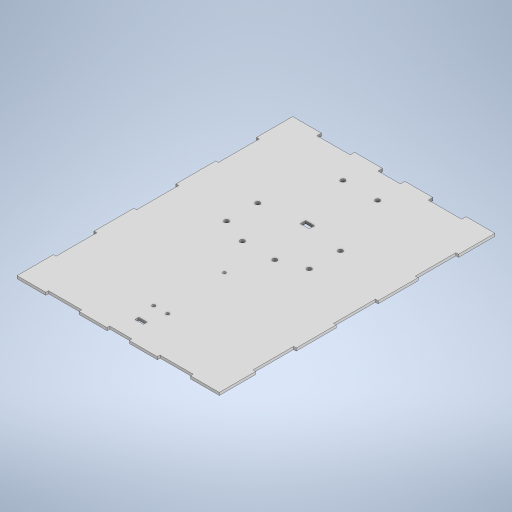
# Autodesk Inventor part: totalPart
Saved by Autodesk Inventor 2023 (Build 270158000, 158)
## iProperties
Created: 2022-11-20
Part Number: totalPart
Material: Generic
Document SubType Name: Modeling
Designer: ADMIN
Density: 1 g/cm^3
Appearance: Default
Author: ADMIN
Autodesk Inventor part; units mm, degrees
ref_plane "YZ Plane" through (0, 0, 0) normal (1, 0, 0) x (0, 1, 0)
ref_plane "XZ Plane" through (0, 0, 0) normal (0, 1, 0) x (-1, 0, 0)
ref_plane "XY Plane" through (0, 0, 0) normal (0, 0, 1) x (1, 0, 0)
sketch "Sketch1" plane through (0, 0, 0) normal (0, 1, 0) x (-1, 0, 0)
  line L0 (128.8824, 62.1664) -> (128.8824, -237.8336)
  line L1 (48.8824, 24.5697) -> (45.8824, 24.5697)
  line L2 (48.8824, -65.4156) -> (45.8824, -65.4156)
  line L3 (48.8824, -20.7764) -> (45.8824, -20.7764)
  line L4 (48.8824, -202.2369) -> (45.8824, -202.2369)
  line L5 (48.8824, -112.2516) -> (45.8824, -112.2516)
  line L6 (48.8824, -156.8908) -> (45.8824, -156.8908)
  line L7 (48.8824, 24.5697) -> (48.8824, 62.1664)
  line L8 (48.8824, 24.5697) -> (48.8824, 65.1664)
  line L9 (48.8824, -65.4156) -> (48.8824, -20.7764)
  line L10 (48.8824, -65.4156) -> (48.8824, -20.7764)
  line L11 (48.8824, -237.8336) -> (48.8824, -202.2369)
  line L12 (48.8824, -156.8908) -> (48.8824, -112.2516)
  line L13 (48.8824, -242.8336) -> (48.8824, -202.2369)
  line L14 (48.8824, -156.8908) -> (48.8824, -112.2516)
  line L15 (45.8824, -20.7764) -> (45.8824, 24.5697)
  line L16 (45.8824, -202.2369) -> (45.8824, -156.8908)
  line L17 (45.8824, -112.2516) -> (45.8824, -65.4156)
  line L18 (-177.1176, 24.5697) -> (-174.1176, 24.5697)
  line L19 (-177.1176, -65.4156) -> (-174.1176, -65.4156)
  line L20 (-177.1176, -20.7764) -> (-174.1176, -20.7764)
  line L21 (-177.1176, -202.2369) -> (-174.1176, -202.2369)
  line L22 (-177.1176, -156.8908) -> (-174.1176, -156.8908)
  line L23 (-177.1176, -112.2516) -> (-174.1176, -112.2516)
  line L24 (-177.1176, 65.1664) -> (-177.1176, 24.5697)
  line L25 (-174.1176, 24.5697) -> (-174.1176, -20.7764)
  line L26 (-177.1176, -20.7764) -> (-177.1176, -65.4156)
  line L27 (-174.1176, -65.4156) -> (-174.1176, -112.2516)
  line L28 (-174.1176, -156.8908) -> (-174.1176, -202.2369)
  line L29 (-177.1176, -112.2516) -> (-177.1176, -156.8908)
  line L30 (-177.1176, -202.2369) -> (-177.1176, -242.8336)
  line L31 (48.8824, -237.8336) -> (48.8824, -242.8336)
  line L32 (128.8824, -242.8336) -> (128.8824, -237.8336)
  line L33 (48.8824, -242.8336) -> (63.8824, -242.8336)
  line L34 (63.8824, -242.8336) -> (63.8824, -237.8336)
  line L35 (63.8824, -237.8336) -> (78.8824, -237.8336)
  line L36 (78.8824, -237.8336) -> (78.8824, -242.8336)
  line L37 (113.8824, -242.8336) -> (113.8824, -237.8336)
  line L38 (98.8824, -237.8336) -> (98.8824, -242.8336)
  line L39 (128.8824, -242.8336) -> (113.8824, -242.8336)
  line L40 (113.8824, -237.8336) -> (98.8824, -237.8336)
  line L41 (78.8824, -237.8336) -> (63.8824, -237.8336)
  line L42 (98.8824, -242.8336) -> (78.8824, -242.8336)
  line L43 (63.8824, -242.8336) -> (48.8824, -242.8336)
  line L44 (63.8824, 65.1664) -> (63.8824, 62.1664)
  line L45 (78.8824, 62.1664) -> (78.8824, 65.1664)
  line L46 (98.8824, 62.1664) -> (98.8824, 65.1664)
  line L47 (113.8824, 65.1664) -> (113.8824, 62.1664)
  line L48 (128.8824, 62.1664) -> (128.8824, 65.1664)
  line L49 (48.8824, 65.1664) -> (63.8824, 65.1664)
  line L50 (63.8824, 62.1664) -> (78.8824, 62.1664)
  line L51 (98.8824, 62.1664) -> (113.8824, 62.1664)
  line L52 (78.8824, 65.1664) -> (98.8824, 65.1664)
  line L53 (113.8824, 65.1664) -> (128.8824, 65.1664)
  line L54 (-174.1176, 145.1664) -> (45.8824, 145.1664)
  line L55 (16.7044, 65.1664) -> (16.7044, 62.1664)
  line L56 (-20.3174, 65.1664) -> (-20.3174, 62.1664)
  line L57 (-51.677, 65.1664) -> (-51.677, 62.1664)
  line L58 (-144.9395, 65.1664) -> (-144.9395, 62.1664)
  line L59 (-107.9177, 65.1664) -> (-107.9177, 62.1664)
  line L60 (-76.5581, 65.1664) -> (-76.5581, 62.1664)
  line L61 (48.8824, 65.1664) -> (16.7044, 65.1664)
  line L62 (-64.1176, 62.1664) -> (-51.677, 62.1664)
  line L63 (-20.3174, 62.1664) -> (16.7044, 62.1664)
  line L64 (16.7044, 62.1664) -> (-20.3174, 62.1664)
  line L65 (-20.3174, 65.1664) -> (-51.677, 65.1664)
  line L66 (-51.677, 62.1664) -> (-76.5581, 62.1664)
  line L67 (-107.9177, 62.1664) -> (-144.9395, 62.1664)
  line L68 (-64.1176, 62.1664) -> (-76.5581, 62.1664)
  line L69 (-76.5581, 65.1664) -> (-107.9177, 65.1664)
  line L70 (-144.9395, 65.1664) -> (-177.1176, 65.1664)
  line L71 (16.7044, -242.8336) -> (16.7044, -237.8336)
  line L72 (-20.3174, -242.8336) -> (-20.3174, -237.8336)
  line L73 (-51.677, -242.8336) -> (-51.677, -237.8336)
  line L74 (-144.9395, -242.8336) -> (-144.9395, -237.8336)
  line L75 (-107.9177, -242.8336) -> (-107.9177, -237.8336)
  line L76 (-76.5581, -242.8336) -> (-76.5581, -237.8336)
  line L77 (-177.1176, -242.8336) -> (-144.9395, -242.8336)
  line L78 (-144.9395, -237.8336) -> (-107.9177, -237.8336)
  line L79 (-107.9177, -242.8336) -> (-76.5581, -242.8336)
  line L80 (-76.5581, -237.8336) -> (-51.677, -237.8336)
  line L81 (-51.677, -242.8336) -> (-20.3174, -242.8336)
  line L82 (16.7044, -242.8336) -> (48.8824, -242.8336)
  line L83 (-20.3174, -237.8336) -> (16.7044, -237.8336)
  line L84 (63.8824, -237.8336) -> (75.0605, -237.8336)
  line L85 (48.8824, 80.1664) -> (48.8824, 95.1664)
  line L86 (48.8824, 95.1664) -> (45.8824, 95.1664)
  line L87 (48.8824, 80.1664) -> (45.8824, 80.1664)
  line L88 (48.8824, 115.1664) -> (45.8824, 115.1664)
  line L89 (48.8824, 130.1664) -> (45.8824, 130.1664)
  line L90 (-177.1176, 95.1664) -> (-174.1176, 95.1664)
  line L91 (-177.1176, 80.1664) -> (-174.1176, 80.1664)
  line L92 (-177.1176, 115.1664) -> (-174.1176, 115.1664)
  line L93 (-177.1176, 130.1664) -> (-174.1176, 130.1664)
  line L94 (45.8824, 80.1664) -> (45.8824, 65.1664)
  line L95 (48.8824, 115.1664) -> (48.8824, 130.1664)
  line L96 (45.8824, 145.1664) -> (45.8824, 130.1664)
  line L97 (45.8824, 115.1664) -> (45.8824, 95.1664)
  line L98 (-174.1176, 65.1664) -> (-174.1176, 80.1664)
  line L99 (-174.1176, 95.1664) -> (-174.1176, 115.1664)
  line L100 (-174.1176, 130.1664) -> (-174.1176, 145.1664)
  line L101 (-177.1176, 80.1664) -> (-177.1176, 95.1664)
  line L102 (-177.1176, 115.1664) -> (-177.1176, 130.1664)
  line L103 (-174.1176, -322.8336) -> (45.8824, -322.8336)
  line L104 (48.8824, -257.8336) -> (48.8824, -272.8336)
  line L105 (48.8824, -272.8336) -> (45.8824, -272.8336)
  line L106 (48.8824, -257.8336) -> (45.8824, -257.8336)
  line L107 (48.8824, -292.8336) -> (45.8824, -292.8336)
  line L108 (48.8824, -307.8336) -> (45.8824, -307.8336)
  line L109 (-177.1176, -307.8336) -> (-174.1176, -307.8336)
  line L110 (-177.1176, -292.8336) -> (-174.1176, -292.8336)
  line L111 (-177.1176, -272.8336) -> (-174.1176, -272.8336)
  line L112 (-177.1176, -257.8336) -> (-174.1176, -257.8336)
  line L113 (45.8824, -257.8336) -> (45.8824, -242.8336)
  line L114 (48.8824, -292.8336) -> (48.8824, -307.8336)
  line L115 (45.8824, -322.8336) -> (45.8824, -307.8336)
  line L116 (45.8824, -292.8336) -> (45.8824, -272.8336)
  line L117 (-174.1176, -242.8336) -> (-174.1176, -257.8336)
  line L118 (-174.1176, -272.8336) -> (-174.1176, -292.8336)
  line L119 (-174.1176, -307.8336) -> (-174.1176, -322.8336)
  line L120 (-177.1176, -257.8336) -> (-177.1176, -272.8336)
  line L121 (-177.1176, -292.8336) -> (-177.1176, -307.8336)
  line L122 (-64.1176, 62.1664) -> (-64.1176, 17.1664)
  line L123 (-64.1176, 17.1664) -> (-64.1176, 17.9164)
  line L124 (-64.1176, 17.9164) -> (-56.6176, 17.9164)
  circle A0 centre (-56.6176, 17.9164) radius 1.75
  circle A1 centre (-72.1176, 17.9164) radius 1.75
  line L125 (-68.6972, 41.8347) -> (-59.538, 41.8347)
  line L126 (-59.538, 41.8347) -> (-59.538, 37.4981)
  line L127 (-59.538, 37.4981) -> (-68.6972, 37.4981)
  line L128 (-68.6972, 37.4981) -> (-68.6972, 41.8347)
  line L129 (-68.6972, 41.8347) -> (-59.538, 37.4981) construction
  line L130 (-59.538, 41.8347) -> (-68.6972, 37.4981) construction
  circle A2 centre (-64.1176, -53.5615) radius 1.6
  line L131 (-69.1176, -149.3399) -> (-59.1176, -149.3399)
  line L132 (-59.1176, -149.3399) -> (-59.1176, -143.3399)
  line L133 (-59.1176, -143.3399) -> (-69.1176, -143.3399)
  line L134 (-69.1176, -143.3399) -> (-69.1176, -149.3399)
  line L135 (-69.1176, -149.3399) -> (-59.1176, -143.3399) construction
  line L136 (-59.1176, -149.3399) -> (-69.1176, -143.3399) construction
  circle A3 centre (-107.9177, -104.5303) radius 2.5
  circle A4 centre (-107.9177, -139.4281) radius 2.5
  circle A5 centre (-15.5025, -104.5303) radius 2.5
  circle A6 centre (-15.5025, -139.4281) radius 2.5
  circle A7 centre (-79.8847, -94.0776) radius 2.5
  circle A8 centre (-43.6456, -94.0776) radius 2.5
  circle A9 centre (-79.8847, -208.9633) radius 2.5
  circle A10 centre (-41.1456, -208.9633) radius 2.5
  point P0 (0, 0)
  point P1 (-20.3174, -239.8336)
  point P2 (-51.677, -239.8336)
  point P3 (-107.9177, -239.8336)
  point P4 (-76.5581, -239.8336)
  point P5 (16.7044, -239.8336)
  point P6 (-144.9395, -239.8336)
  point P7 (-126.4286, -237.8336)
  point P8 (-126.4286, 62.1664)
  point P9 (-161.0285, 65.1664)
  point P10 (-174.1176, -179.5638)
  point P11 (-64.1176, 39.6664)
  point P12 (-64.1176, -146.3399)
  dimension "d0" = 226
  dimension "d1" = 308
  dimension "d6" = 80
  dimension "d7" = 15
  dimension "d8" = 15
  dimension "d11" = 300
  dimension "d12" = 15
  dimension "d13" = 15
  dimension "d14" = 80
  dimension "d15" = 220
  dimension "d16" = 5
  dimension "d19" = 45
  dimension "d20" = 0.75
  dimension "d21" = 7.5
  dimension "d22" = 3.5
  dimension "d23" = 3.5
  dimension "d24" = 15.5
  dimension "d25" = 3.2
  dimension "d26" = 10
  dimension "d27" = 6
  dimension "d28" = 5
  dimension "d29" = 5
  dimension "d30" = 5
  dimension "d31" = 5
  dimension "d32" = 5
  dimension "d33" = 5
  dimension "d34" = 5
  dimension "d35" = 5
  constraints: 274 end point, 72 parallel, 65 perpendicular, 17 horizontal, 11 centre point, 10 point on line, 9 midpoint, 4 vertical, 1 coincident, 1 collinear
  measures "d0" distance of L13.start L30.end
  measures "d1" distance of L30.end L24.start
  measures "d6" distance of L0.end L11.start
  measures "d7" distance of L13.start L33.end
  measures "d8" distance of L34.end L35.end
  measures "d11" distance of point (-126.429, -237.834) point (-126.429, 62.166)
  measures "d12" distance of L8.end L85.start
  measures "d13" distance of L85.start L85.end
  measures "d14" distance from line of point (-161.029, 65.166) L54
  measures "d15" distance from line of point (-174.118, -179.564) L16
  measures "d16" distance of L71.start L71.end
  measures "d19" distance of L62.start L122.end
  measures "d20" distance of L122.end L123.end
  measures "d21" distance of L123.end L124.end
  measures "d22" diameter of A0
  measures "d23" diameter of A1
  measures "d24" distance of A1.centre L124.end
  measures "d25" diameter of A2
  measures "d26" distance of L133.end L132.end
  measures "d27" distance of L132.end L131.end
  measures "d28" diameter of A3
  measures "d29" diameter of A4
  measures "d30" diameter of A5
  measures "d31" diameter of A6
  measures "d32" diameter of A7
  measures "d33" diameter of A8
  measures "d34" diameter of A9
  measures "d35" diameter of A10
extrude "Extrusion1" add sketch "Sketch1" along normal blind 3 contours L8 L7 L1 L15 L3 L9 L2 L17 L5 L12 L6 L16 L4 L11 L13 L82 L71 L83 L72 L81 L73 L80 L76 L79 L75 L78 L74 L77 L30 L21 L28 L22 L29 L23 L27 L19 L26 L20 L25 L18 L24 L70 L58 L67 L59 L69 L60 L66 L62 L57 L65 L56 L63 L55 L61
body "Solid1"
